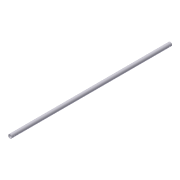
# Autodesk Inventor part: FE-00005-04
Saved by Autodesk Inventor 2012 (Build 160160000, 160)
## iProperties
Company: FIRST
Created: 2008-05-25
Part Number: FE-00005-04
Document SubType Name: Modeling
Designer: dfoster
Density: 1 g/cm^3
Description: Top Rail
Mass: 788.819 g
Surface Area: 4432.25 cm^2
Volume: 788.819 cm^3
Material: Default
Title: Top Rail
Author: dfoster
Autodesk Inventor part; units mm, degrees
ref_plane "XZ Plane" through (0, 0, 0) normal (0, 1, 0) x (-1, 0, 0)
sketch "Sketch1" plane through (0, 0, 0) normal (0, 0, 1) x (1, 0, 0)
  circle A0 centre (0, 0) radius 21.0312
  circle A1 centre (0, 0) radius 17.4625
  dimension "d0" = 42.0624
  dimension "d1" = 34.925
  constraints: 2 centre point, 1 coincident
  measures "d0" diameter of A0
  measures "d1" diameter of A1
extrude "Extrusion1" add sketch "Sketch1" along normal blind 1828.8
ref_plane "Work Plane1" through (0, 0, 0) normal (1, 0, 0) x (0, 0, 1)
sketch "Sketch2" plane through (0, 0, 0) normal (1, 0, 0) x (0, 0, 1)
  circle A0 centre (31.75, 0) radius 3.175
  line L0 (-365.76, 0) -> (2194.56, 0) projected
  line L1 (0, 21.0312) -> (0, -21.0312) projected
  dimension "d5" = 6.35
  dimension "d6" = 31.75
  constraints: 1 centre point, 1 point on line
  measures "d5" diameter of A0
  measures "d6" distance from line of L1 A0.centre
extrude "Extrusion2" cut sketch "Sketch2" along normal blind 381
pattern_linear "Rectangular Pattern1" count 2 spacing 50.8 along (0, 0, 1) of "Extrusion2"
ref_plane "Work Plane2" through (0, 0, 914.4) normal (0, 0, 1) x (1, 0, 0)
mirror "Mirror1" about plane through (0, 0, 914.4) normal (0, 0, 1) of "Extrusion2", "Rectangular Pattern1"
body "Solid1"
